Autodesk Fusion 360 part; units mm, degrees
(part 2 of 3)
  line L889 (-65.0001, -30.25) -> (-65.0001, -32.25)
  line L890 (-62.5001, -30.25) -> (-62.5001, -32.25)
  line L891 (-27.5001, -35.25) -> (-27.5001, -37.25)
  line L892 (-32.5001, -39.75) -> (-30.5001, -39.75)
  line L893 (-30.5001, -32.75) -> (-32.5001, -32.75)
  line L894 (-55.5001, -37.25) -> (-55.5001, -35.25)
  line L895 (-32.5001, -32.25) -> (-30.5001, -32.25)
  line L896 (-53.0001, -40.25) -> (-55.0001, -40.25)
  line L897 (-30.5001, -34.75) -> (-30.5001, -32.75)
  line L898 (-30.5001, -32.25) -> (-30.5001, -30.25)
  line L899 (-72.5001, -37.75) -> (-72.5001, -39.75)
  line L900 (-32.5001, -30.25) -> (-32.5001, -32.25)
  line L901 (-28.0001, -37.25) -> (-28.0001, -35.25)
  line L902 (-38.0001, -34.75) -> (-38.0001, -32.75)
  line L903 (-55.0001, -37.25) -> (-53.0001, -37.25)
  line L904 (-55.0001, -37.75) -> (-55.0001, -39.75)
  line L905 (-30.0001, -37.25) -> (-28.0001, -37.25)
  line L906 (-72.5001, -39.75) -> (-70.5001, -39.75)
  line L907 (-15.0001, -37.75) -> (-15.0001, -39.75)
  line L908 (-30.5001, -30.25) -> (-32.5001, -30.25)
  line L909 (-72.5001, -34.75) -> (-70.5001, -34.75)
  line L910 (-53.0001, -30.25) -> (-55.0001, -30.25)
  line L911 (-12.5001, -32.25) -> (-10.5001, -32.25)
  line L912 (-40.5001, -32.75) -> (-42.5001, -32.75)
  line L913 (-53.0001, -42.25) -> (-53.0001, -40.25)
  line L914 (-53.0001, -39.75) -> (-53.0001, -37.75)
  line L915 (-30.0001, -37.75) -> (-30.0001, -39.75)
  line L916 (-55.5001, -42.25) -> (-55.5001, -40.25)
  line L917 (-15.5001, -39.75) -> (-15.5001, -37.75)
  line L918 (-55.0001, -39.75) -> (-53.0001, -39.75)
  line L919 (-53.0001, -35.25) -> (-55.0001, -35.25)
  line L920 (-40.5001, -30.25) -> (-42.5001, -30.25)
  line L921 (-27.5001, -37.75) -> (-27.5001, -39.75)
  line L922 (-72.5001, -37.25) -> (-70.5001, -37.25)
  line L923 (-40.5001, -35.25) -> (-42.5001, -35.25)
  line L924 (-32.5001, -32.75) -> (-32.5001, -34.75)
  line L925 (-30.5001, -35.25) -> (-32.5001, -35.25)
  line L926 (-70.5001, -32.75) -> (-72.5001, -32.75)
  line L927 (-72.5001, -32.25) -> (-70.5001, -32.25)
  line L928 (-53.0001, -37.75) -> (-55.0001, -37.75)
  line L929 (-12.5001, -34.75) -> (-10.5001, -34.75)
  line L930 (-55.0001, -30.25) -> (-55.0001, -32.25)
  line L931 (-40.5001, -32.25) -> (-40.5001, -30.25)
  line L932 (-40.5001, -34.75) -> (-40.5001, -32.75)
  line L933 (-13.0001, -39.75) -> (-13.0001, -37.75)
  line L934 (-72.5001, -32.75) -> (-72.5001, -34.75)
  line L935 (-55.0001, -34.75) -> (-53.0001, -34.75)
  line L936 (-53.0001, -37.25) -> (-53.0001, -35.25)
  line L937 (-32.5001, -34.75) -> (-30.5001, -34.75)
  line L938 (-53.0001, -32.25) -> (-53.0001, -30.25)
  line L939 (-28.0001, -39.75) -> (-28.0001, -37.75)
  line L940 (-30.0001, -35.25) -> (-30.0001, -37.25)
  line L941 (-30.0001, -32.25) -> (-28.0001, -32.25)
  line L942 (-30.0001, -32.75) -> (-30.0001, -34.75)
  line L943 (-40.0001, -32.75) -> (-40.0001, -34.75)
  line L944 (-10.5001, -37.75) -> (-12.5001, -37.75)
  line L945 (-32.5001, -35.25) -> (-32.5001, -37.25)
  line L946 (-30.0001, -30.25) -> (-30.0001, -32.25)
  line L947 (-42.5001, -34.75) -> (-40.5001, -34.75)
  line L948 (-55.0001, -40.25) -> (-55.0001, -42.25)
  line L949 (-55.0001, -42.25) -> (-53.0001, -42.25)
  line L950 (-70.5001, -37.75) -> (-72.5001, -37.75)
  line L951 (-55.5001, -39.75) -> (-55.5001, -37.75)
  line L952 (-55.0001, -35.25) -> (-55.0001, -37.25)
  line L953 (-15.0001, -32.25) -> (-13.0001, -32.25)
  line L954 (-75.5001, -40.25) -> (-77.5001, -40.25)
  line L955 (-53.0001, -34.75) -> (-53.0001, -32.75)
  line L956 (-77.5001, -42.25) -> (-75.5001, -42.25)
  line L957 (-53.0001, -32.75) -> (-55.0001, -32.75)
  line L958 (-78.0001, -42.25) -> (-78.0001, -40.25)
  line L959 (-25.5001, -34.75) -> (-25.5001, -32.75)
  line L960 (-55.5001, -32.25) -> (-55.5001, -30.25)
  line L961 (-67.5001, -32.75) -> (-67.5001, -34.75)
  line L962 (-27.5001, -42.25) -> (-25.5001, -42.25)
  line L963 (-33.0001, -37.25) -> (-33.0001, -35.25)
  line L964 (-40.0001, -32.25) -> (-38.0001, -32.25)
  line L965 (-38.0001, -32.25) -> (-38.0001, -30.25)
  line L966 (-70.0001, -32.75) -> (-70.0001, -34.75)
  line L967 (-55.0001, -32.75) -> (-55.0001, -34.75)
  line L968 (-20.5001, -37.75) -> (-22.5001, -37.75)
  line L969 (-28.0001, -32.25) -> (-28.0001, -30.25)
  line L970 (-13.0001, -30.25) -> (-15.0001, -30.25)
  line L971 (-25.0001, -32.75) -> (-25.0001, -34.75)
  line L972 (-70.5001, -35.25) -> (-72.5001, -35.25)
  line L973 (-55.5001, -34.75) -> (-55.5001, -32.75)
  line L974 (-27.5001, -30.25) -> (-27.5001, -32.25)
  line L975 (-72.5001, -30.25) -> (-72.5001, -32.25)
  line L976 (-13.0001, -32.75) -> (-15.0001, -32.75)
  line L977 (-20.5001, -35.25) -> (-22.5001, -35.25)
  line L978 (-15.0001, -30.25) -> (-15.0001, -32.25)
  line L979 (-35.0001, -42.25) -> (-33.0001, -42.25)
  line L980 (-72.5001, -35.25) -> (-72.5001, -37.25)
  line L981 (-13.0001, -32.25) -> (-13.0001, -30.25)
  line L982 (-12.5001, -32.75) -> (-12.5001, -34.75)
  line L983 (-70.0001, -30.25) -> (-70.0001, -32.25)
  line L984 (-27.5001, -32.75) -> (-27.5001, -34.75)
  line L985 (-40.0001, -30.25) -> (-40.0001, -32.25)
  line L986 (-35.5001, -40.25) -> (-37.5001, -40.25)
  line L987 (-33.0001, -40.25) -> (-35.0001, -40.25)
  line L988 (-28.0001, -34.75) -> (-28.0001, -32.75)
  line L989 (-70.5001, -30.25) -> (-72.5001, -30.25)
  line L990 (-33.0001, -42.25) -> (-33.0001, -40.25)
  line L991 (-37.5001, -40.25) -> (-37.5001, -42.25)
  line L992 (-40.5001, -37.25) -> (-40.5001, -35.25)
  line L993 (-22.5001, -34.75) -> (-20.5001, -34.75)
  line L994 (-37.5001, -42.25) -> (-35.5001, -42.25)
  line L995 (-55.0001, -32.25) -> (-53.0001, -32.25)
  line L996 (-15.5001, -34.75) -> (-15.5001, -32.75)
  line L997 (-30.5001, -37.25) -> (-30.5001, -35.25)
  line L998 (-38.0001, -30.25) -> (-40.0001, -30.25)
  line L999 (-35.5001, -42.25) -> (-35.5001, -40.25)
  line L1000 (-68.0001, -34.75) -> (-68.0001, -32.75)
  line L1001 (-15.5001, -32.25) -> (-15.5001, -30.25)
  line L1002 (-22.5001, -39.75) -> (-20.5001, -39.75)
  line L1003 (-35.0001, -40.25) -> (-35.0001, -42.25)
  line L1004 (-77.5001, -40.25) -> (-77.5001, -42.25)
  line L1005 (-42.5001, -32.25) -> (-40.5001, -32.25)
  line L1006 (-12.5001, -30.25) -> (-12.5001, -32.25)
  line L1007 (-47.5001, -37.75) -> (-47.5001, -39.75)
  line L1008 (-43.0001, -39.75) -> (-43.0001, -37.75)
  line L1009 (-45.0001, -37.75) -> (-45.0001, -39.75)
  line L1010 (-67.5001, -35.25) -> (-67.5001, -37.25)
  line L1011 (-75.5001, -35.25) -> (-77.5001, -35.25)
  line L1012 (-57.5001, -35.25) -> (-57.5001, -37.25)
  line L1013 (-57.5001, -37.25) -> (-55.5001, -37.25)
  line L1014 (-25.5001, -37.75) -> (-27.5001, -37.75)
  line L1015 (-35.0001, -34.75) -> (-33.0001, -34.75)
  line L1016 (-78.0001, -34.75) -> (-78.0001, -32.75)
  line L1017 (-35.5001, -32.25) -> (-35.5001, -30.25)
  line L1018 (-35.5001, -34.75) -> (-35.5001, -32.75)
  line L1019 (-60.0001, -40.25) -> (-60.0001, -42.25)
  line L1020 (-57.5001, -34.75) -> (-55.5001, -34.75)
  line L1021 (-55.5001, -35.25) -> (-57.5001, -35.25)
  line L1022 (-78.0001, -39.75) -> (-78.0001, -37.75)
  line L1023 (-37.5001, -30.25) -> (-37.5001, -32.25)
  line L1024 (-65.5001, -35.25) -> (-67.5001, -35.25)
  line L1025 (-55.5001, -37.75) -> (-57.5001, -37.75)
  line L1026 (-77.5001, -39.75) -> (-75.5001, -39.75)
  line L1027 (-25.5001, -37.25) -> (-25.5001, -35.25)
  line L1028 (-35.5001, -30.25) -> (-37.5001, -30.25)
  line L1029 (-67.5001, -34.75) -> (-65.5001, -34.75)
  line L1030 (-58.0001, -37.75) -> (-60.0001, -37.75)
  line L1031 (-60.0001, -39.75) -> (-58.0001, -39.75)
  line L1032 (-35.5001, -35.25) -> (-37.5001, -35.25)
  line L1033 (-55.5001, -32.75) -> (-57.5001, -32.75)
  line L1034 (-57.5001, -40.25) -> (-57.5001, -42.25)
  line L1035 (-35.0001, -37.75) -> (-35.0001, -39.75)
  line L1036 (-37.5001, -37.25) -> (-35.5001, -37.25)
  line L1037 (-37.5001, -32.75) -> (-37.5001, -34.75)
  line L1038 (-33.0001, -35.25) -> (-35.0001, -35.25)
  line L1039 (-60.0001, -37.25) -> (-58.0001, -37.25)
  line L1040 (-60.5001, -42.25) -> (-60.5001, -40.25)
  line L1041 (-57.5001, -37.75) -> (-57.5001, -39.75)
  line L1042 (-77.5001, -37.75) -> (-77.5001, -39.75)
  line L1043 (-33.0001, -32.75) -> (-35.0001, -32.75)
  line L1044 (-37.5001, -39.75) -> (-35.5001, -39.75)
  line L1045 (-73.0001, -32.75) -> (-75.0001, -32.75)
  line L1046 (-58.0001, -42.25) -> (-58.0001, -40.25)
  line L1047 (-27.5001, -37.25) -> (-25.5001, -37.25)
  line L1048 (-68.0001, -37.25) -> (-68.0001, -35.25)
  line L1049 (-60.5001, -39.75) -> (-60.5001, -37.75)
  line L1050 (-37.5001, -34.75) -> (-35.5001, -34.75)
  line L1051 (-37.5001, -32.25) -> (-35.5001, -32.25)
  line L1052 (-75.0001, -34.75) -> (-73.0001, -34.75)
  line L1053 (-60.0001, -37.75) -> (-60.0001, -39.75)
  line L1054 (-77.5001, -37.25) -> (-75.5001, -37.25)
  line L1055 (-35.5001, -39.75) -> (-35.5001, -37.75)
  line L1056 (-67.5001, -37.25) -> (-65.5001, -37.25)
  line L1057 (-33.0001, -34.75) -> (-33.0001, -32.75)
  line L1058 (-75.5001, -30.25) -> (-77.5001, -30.25)
  line L1059 (-75.0001, -32.75) -> (-75.0001, -34.75)
  line L1060 (-35.0001, -32.75) -> (-35.0001, -34.75)
  line L1061 (-78.0001, -32.25) -> (-78.0001, -30.25)
  line L1062 (-58.0001, -40.25) -> (-60.0001, -40.25)
  line L1063 (-75.5001, -32.75) -> (-77.5001, -32.75)
  line L1064 (-77.5001, -30.25) -> (-77.5001, -32.25)
  line L1065 (-75.5001, -37.75) -> (-77.5001, -37.75)
  line L1066 (-58.0001, -39.75) -> (-58.0001, -37.75)
  line L1067 (-60.0001, -42.25) -> (-58.0001, -42.25)
  line L1068 (-65.5001, -37.75) -> (-67.5001, -37.75)
  line L1069 (-73.0001, -35.25) -> (-75.0001, -35.25)
  line L1070 (-77.5001, -32.25) -> (-75.5001, -32.25)
  line L1071 (-58.0001, -32.25) -> (-58.0001, -30.25)
  line L1072 (-58.0001, -30.25) -> (-60.0001, -30.25)
  line L1073 (-20.0001, -32.25) -> (-18.0001, -32.25)
  line L1074 (-20.0001, -39.75) -> (-18.0001, -39.75)
  line L1075 (-18.0001, -42.25) -> (-18.0001, -40.25)
  line L1076 (-17.5001, -40.25) -> (-17.5001, -42.25)
  line L1077 (-17.5001, -30.25) -> (-17.5001, -32.25)
  line L1078 (-20.5001, -34.75) -> (-20.5001, -32.75)
  line L1079 (-75.0001, -30.25) -> (-75.0001, -32.25)
  line L1080 (-60.5001, -37.25) -> (-60.5001, -35.25)
  line L1081 (-35.0001, -32.25) -> (-33.0001, -32.25)
  line L1082 (-18.0001, -34.75) -> (-18.0001, -32.75)
  line L1083 (-17.5001, -37.75) -> (-17.5001, -39.75)
  line L1084 (-20.5001, -32.25) -> (-20.5001, -30.25)
  line L1085 (-20.0001, -42.25) -> (-18.0001, -42.25)
  line L1086 (-18.0001, -32.75) -> (-20.0001, -32.75)
  line L1087 (-35.0001, -30.25) -> (-35.0001, -32.25)
  line L1088 (-33.0001, -30.25) -> (-35.0001, -30.25)
  line L1089 (-58.0001, -35.25) -> (-60.0001, -35.25)
  line L1090 (-33.0001, -32.25) -> (-33.0001, -30.25)
  line L1091 (-73.0001, -30.25) -> (-75.0001, -30.25)
  line L1092 (-57.5001, -32.25) -> (-55.5001, -32.25)
  line L1093 (-55.5001, -40.25) -> (-57.5001, -40.25)
  line L1094 (-57.5001, -30.25) -> (-57.5001, -32.25)
  line L1095 (-58.0001, -37.25) -> (-58.0001, -35.25)
  line L1096 (-17.5001, -32.75) -> (-17.5001, -34.75)
  line L1097 (-60.0001, -32.25) -> (-58.0001, -32.25)
  line L1098 (-60.5001, -32.25) -> (-60.5001, -30.25)
  line L1099 (-75.0001, -32.25) -> (-73.0001, -32.25)
  line L1100 (-55.5001, -30.25) -> (-57.5001, -30.25)
  line L1101 (-60.0001, -32.75) -> (-60.0001, -34.75)
  line L1102 (-58.0001, -32.75) -> (-60.0001, -32.75)
  line L1103 (-58.0001, -34.75) -> (-58.0001, -32.75)
  line L1104 (-20.0001, -37.75) -> (-20.0001, -39.75)
  line L1105 (-18.0001, -39.75) -> (-18.0001, -37.75)
  line L1106 (-20.5001, -39.75) -> (-20.5001, -37.75)
  line L1107 (-77.5001, -34.75) -> (-75.5001, -34.75)
  line L1108 (-57.5001, -42.25) -> (-55.5001, -42.25)
  line L1109 (-60.0001, -34.75) -> (-58.0001, -34.75)
  line L1110 (-57.5001, -32.75) -> (-57.5001, -34.75)
  line L1111 (-20.0001, -32.75) -> (-20.0001, -34.75)
  line L1112 (-60.5001, -34.75) -> (-60.5001, -32.75)
  line L1113 (-57.5001, -39.75) -> (-55.5001, -39.75)
  line L1114 (-60.0001, -30.25) -> (-60.0001, -32.25)
  line L1115 (-60.0001, -35.25) -> (-60.0001, -37.25)
  line L1116 (-77.5001, -32.75) -> (-77.5001, -34.75)
  line L1117 (-78.0001, -40.25) -> (-80.0001, -40.25)
  line L1118 (-62.5001, -40.25) -> (-62.5001, -42.25)
  line L1119 (-20.5001, -42.25) -> (-20.5001, -40.25)
  line L1120 (-18.0001, -30.25) -> (-20.0001, -30.25)
  line L1121 (-75.5001, -34.75) -> (-75.5001, -32.75)
  line L1122 (-65.5001, -42.25) -> (-65.5001, -40.25)
  line L1123 (-75.5001, -42.25) -> (-75.5001, -40.25)
  line L1124 (-65.0001, -42.25) -> (-63.0001, -42.25)
  line L1125 (-17.5001, -35.25) -> (-17.5001, -37.25)
  line L1126 (-20.0001, -37.25) -> (-18.0001, -37.25)
  line L1127 (-70.0001, -37.75) -> (-70.0001, -39.75)
  line L1128 (-20.0001, -30.25) -> (-20.0001, -32.25)
  line L1129 (-75.5001, -39.75) -> (-75.5001, -37.75)
  line L1130 (-18.0001, -35.25) -> (-20.0001, -35.25)
  line L1131 (-73.0001, -37.75) -> (-75.0001, -37.75)
  line L1132 (-18.0001, -37.25) -> (-18.0001, -35.25)
  line L1133 (-20.5001, -37.25) -> (-20.5001, -35.25)
  line L1134 (-68.0001, -40.25) -> (-70.0001, -40.25)
  line L1135 (-75.0001, -40.25) -> (-75.0001, -42.25)
  line L1136 (-80.0001, -32.75) -> (-80.0001, -34.75)
  line L1137 (-70.0001, -40.25) -> (-70.0001, -42.25)
  line L1138 (-70.0001, -37.25) -> (-68.0001, -37.25)
  line L1139 (-75.0001, -42.25) -> (-73.0001, -42.25)
  line L1140 (-70.5001, -42.25) -> (-70.5001, -40.25)
  line L1141 (-20.0001, -34.75) -> (-18.0001, -34.75)
  line L1142 (-18.0001, -32.25) -> (-18.0001, -30.25)
  line L1143 (-73.0001, -40.25) -> (-75.0001, -40.25)
  line L1144 (-18.0001, -40.25) -> (-20.0001, -40.25)
  line L1145 (-73.0001, -39.75) -> (-73.0001, -37.75)
  line L1146 (-18.0001, -37.75) -> (-20.0001, -37.75)
  line L1147 (-80.0001, -39.75) -> (-78.0001, -39.75)
  line L1148 (-73.0001, -42.25) -> (-73.0001, -40.25)
  line L1149 (-63.0001, -40.25) -> (-65.0001, -40.25)
  line L1150 (-70.0001, -42.25) -> (-68.0001, -42.25)
  line L1151 (-20.0001, -40.25) -> (-20.0001, -42.25)
  line L1152 (-73.0001, -32.25) -> (-73.0001, -30.25)
  line L1153 (-20.0001, -35.25) -> (-20.0001, -37.25)
  line L1154 (-70.0001, -39.75) -> (-68.0001, -39.75)
  line L1155 (-80.0001, -37.75) -> (-80.0001, -39.75)
  line L1156 (-63.0001, -42.25) -> (-63.0001, -40.25)
  line L1157 (-70.5001, -39.75) -> (-70.5001, -37.75)
  line L1158 (-80.0001, -40.25) -> (-80.0001, -42.25)
  line L1159 (-65.0001, -40.25) -> (-65.0001, -42.25)
  line L1160 (-75.0001, -37.25) -> (-73.0001, -37.25)
  line L1161 (-75.0001, -39.75) -> (-73.0001, -39.75)
  line L1162 (-80.0001, -42.25) -> (-78.0001, -42.25)
  line L1163 (-75.0001, -37.75) -> (-75.0001, -39.75)
  line L1164 (-78.0001, -37.25) -> (-78.0001, -35.25)
  line L1165 (-35.0001, -35.25) -> (-35.0001, -37.25)
  line L1166 (-68.0001, -42.25) -> (-68.0001, -40.25)
  line L1167 (-27.5001, -32.25) -> (-25.5001, -32.25)
  line L1168 (-65.5001, -30.25) -> (-67.5001, -30.25)
  line L1169 (-77.5001, -35.25) -> (-77.5001, -37.25)
  line L1170 (-37.5001, -37.75) -> (-37.5001, -39.75)
  line L1171 (-25.5001, -40.25) -> (-27.5001, -40.25)
  line L1172 (-25.0001, -37.75) -> (-25.0001, -39.75)
  line L1173 (-27.5001, -39.75) -> (-25.5001, -39.75)
  line L1174 (-35.0001, -37.25) -> (-33.0001, -37.25)
  line L1175 (-65.5001, -32.75) -> (-67.5001, -32.75)
  line L1176 (-68.0001, -32.25) -> (-68.0001, -30.25)
  line L1177 (-67.5001, -40.25) -> (-67.5001, -42.25)
  line L1178 (-67.5001, -32.25) -> (-65.5001, -32.25)
  line L1179 (-67.5001, -30.25) -> (-67.5001, -32.25)
  line L1180 (-35.0001, -39.75) -> (-33.0001, -39.75)
  line L1181 (-35.5001, -37.75) -> (-37.5001, -37.75)
  line L1182 (-67.5001, -37.75) -> (-67.5001, -39.75)
  line L1183 (-25.5001, -32.75) -> (-27.5001, -32.75)
  line L1184 (-25.0001, -30.25) -> (-25.0001, -32.25)
  line L1185 (-25.5001, -42.25) -> (-25.5001, -40.25)
  line L1186 (-67.5001, -39.75) -> (-65.5001, -39.75)
  line L1187 (-35.5001, -37.25) -> (-35.5001, -35.25)
  line L1188 (-25.0001, -35.25) -> (-25.0001, -37.25)
  line L1189 (-35.5001, -32.75) -> (-37.5001, -32.75)
  line L1190 (-33.0001, -37.75) -> (-35.0001, -37.75)
  line L1191 (-65.5001, -40.25) -> (-67.5001, -40.25)
  line L1192 (-25.5001, -35.25) -> (-27.5001, -35.25)
  line L1193 (-27.5001, -34.75) -> (-25.5001, -34.75)
  line L1194 (-25.5001, -39.75) -> (-25.5001, -37.75)
  line L1195 (-33.0001, -39.75) -> (-33.0001, -37.75)
  line L1196 (-25.5001, -30.25) -> (-27.5001, -30.25)
  line L1197 (-67.5001, -42.25) -> (-65.5001, -42.25)
  line L1198 (-25.5001, -32.25) -> (-25.5001, -30.25)
  line L1199 (-37.5001, -35.25) -> (-37.5001, -37.25)
  line L1200 (-68.0001, -39.75) -> (-68.0001, -37.75)
  line L1201 (-25.0001, -40.25) -> (-25.0001, -42.25)
  line L1202 (-43.0001, -35.25) -> (-45.0001, -35.25)
  line L1203 (-50.0001, -34.75) -> (-48.0001, -34.75)
  line L1204 (-48.0001, -37.75) -> (-50.0001, -37.75)
  line L1205 (-50.5001, -37.25) -> (-50.5001, -35.25)
  line L1206 (-42.5001, -32.75) -> (-42.5001, -34.75)
  line L1207 (-50.5001, -39.75) -> (-50.5001, -37.75)
  line L1208 (-45.5001, -39.75) -> (-45.5001, -37.75)
  line L1209 (-50.0001, -37.25) -> (-48.0001, -37.25)
  line L1210 (-50.0001, -35.25) -> (-50.0001, -37.25)
  line L1211 (-48.0001, -35.25) -> (-50.0001, -35.25)
  line L1212 (-45.0001, -34.75) -> (-43.0001, -34.75)
  line L1213 (-45.0001, -37.25) -> (-43.0001, -37.25)
  line L1214 (-43.0001, -37.25) -> (-43.0001, -35.25)
  line L1215 (-45.5001, -35.25) -> (-47.5001, -35.25)
  line L1216 (-45.5001, -37.25) -> (-45.5001, -35.25)
  line L1217 (-42.5001, -35.25) -> (-42.5001, -37.25)
  line L1218 (-47.5001, -37.25) -> (-45.5001, -37.25)
  line L1219 (-47.5001, -35.25) -> (-47.5001, -37.25)
  line L1220 (-48.0001, -37.25) -> (-48.0001, -35.25)
  line L1221 (-50.0001, -37.75) -> (-50.0001, -39.75)
  line L1222 (-48.0001, -39.75) -> (-48.0001, -37.75)
  line L1223 (-47.5001, -30.25) -> (-47.5001, -32.25)
  line L1224 (-48.0001, -34.75) -> (-48.0001, -32.75)
  line L1225 (-50.0001, -32.75) -> (-50.0001, -34.75)
  line L1226 (-50.5001, -34.75) -> (-50.5001, -32.75)
  line L1227 (-50.0001, -32.25) -> (-48.0001, -32.25)
  line L1228 (-45.0001, -30.25) -> (-45.0001, -32.25)
  line L1229 (-43.0001, -34.75) -> (-43.0001, -32.75)
  line L1230 (-43.0001, -32.25) -> (-43.0001, -30.25)
  line L1231 (-45.0001, -32.25) -> (-43.0001, -32.25)
  line L1232 (-45.5001, -32.25) -> (-45.5001, -30.25)
  line L1233 (-50.5001, -32.25) -> (-50.5001, -30.25)
  line L1234 (-45.5001, -32.75) -> (-47.5001, -32.75)
  line L1235 (-48.0001, -32.25) -> (-48.0001, -30.25)
  line L1236 (-45.5001, -30.25) -> (-47.5001, -30.25)
  line L1237 (-43.0001, -32.75) -> (-45.0001, -32.75)
  line L1238 (-48.0001, -32.75) -> (-50.0001, -32.75)
  line L1239 (-43.0001, -30.25) -> (-45.0001, -30.25)
  line L1240 (-47.5001, -32.25) -> (-45.5001, -32.25)
  line L1241 (-50.0001, -30.25) -> (-50.0001, -32.25)
  line L1242 (-48.0001, -30.25) -> (-50.0001, -30.25)
  line L1243 (-42.5001, -30.25) -> (-42.5001, -32.25)
  line L1244 (-47.5001, -32.75) -> (-47.5001, -34.75)
  line L1245 (-45.5001, -34.75) -> (-45.5001, -32.75)
  dimension "d443" = 3.0001
  dimension "d445" = 2.9999
  dimension "d446" = 1.75
  constraint horizontal L9
  constraint vertical L6
  constraint horizontal L7
  constraint vertical L8
  constraint horizontal L10
  constraint vertical L11
  constraint horizontal L12
  constraint vertical L13
  constraint horizontal L16
  constraint vertical L17
  constraint horizontal L14
  constraint vertical L15
  constraint horizontal L21
  constraint vertical L20
  constraint horizontal L18
  constraint vertical L19
  constraint horizontal L24
  constraint vertical L25
  constraint horizontal L22
  constraint vertical L23
  constraint horizontal L32
  constraint vertical L26
  constraint horizontal L33
  constraint vertical L29
  constraint horizontal L39
  constraint vertical L43
  constraint horizontal L41
  constraint vertical L40
  constraint horizontal L37
  constraint vertical L42
  constraint horizontal L38
  constraint vertical L35
  constraint horizontal L28
  constraint vertical L34
  constraint horizontal L45
  constraint vertical L27
  constraint horizontal L36
  constraint vertical L31
  constraint horizontal L30
  constraint vertical L44
  constraint horizontal L60
  constraint vertical L61
  constraint horizontal L84
  constraint vertical L81
  constraint horizontal L66
  constraint vertical L72
  constraint horizontal L85
  constraint vertical L64
  constraint horizontal L51
  constraint vertical L65
  constraint horizontal L58
  constraint vertical L47
  constraint horizontal L62
  constraint vertical L68
  constraint horizontal L63
  constraint vertical L71
  constraint horizontal L55
  constraint vertical L73
  constraint horizontal L78
  constraint vertical L79
  constraint horizontal L49
  constraint vertical L46
  constraint horizontal L80
  constraint vertical L57
  constraint horizontal L69
  constraint vertical L67
  constraint horizontal L59
  constraint vertical L56
  constraint horizontal L50
  constraint vertical L54
  constraint horizontal L76
  constraint vertical L48
  constraint horizontal L77
  constraint vertical L83
  constraint horizontal L75
  constraint vertical L82
  constraint horizontal L70
  constraint vertical L53
  constraint horizontal L74
  constraint vertical L52
  constraint horizontal L89
  constraint vertical L151
  constraint horizontal L102
  constraint vertical L86
  constraint horizontal L155
  constraint vertical L164
  constraint horizontal L109
  constraint vertical L146
  constraint horizontal L145
  constraint vertical L108
  constraint horizontal L91
  constraint vertical L126
  constraint horizontal L95
  constraint vertical L152
  constraint horizontal L103
  constraint vertical L100
  constraint horizontal L101
  constraint vertical L88
  constraint horizontal L99
  constraint vertical L96
  constraint horizontal L156
  constraint vertical L122
  constraint horizontal L147
  constraint vertical L90
  constraint horizontal L150
  constraint vertical L87
  constraint horizontal L148
  constraint vertical L98
  constraint horizontal L133
  constraint vertical L104
  constraint horizontal L163
  constraint vertical L123
  constraint horizontal L94
  constraint vertical L143
  constraint horizontal L160
  constraint vertical L92
  constraint horizontal L134
  constraint vertical L107
  constraint horizontal L153
  constraint vertical L97
  constraint horizontal L105
  constraint vertical L119
  constraint horizontal L131
  constraint vertical L110
  constraint horizontal L154
  constraint vertical L132
  constraint horizontal L162
  constraint vertical L93
  constraint horizontal L149
  constraint vertical L124
  constraint horizontal L140
  constraint vertical L125
  constraint horizontal L139
  constraint vertical L135
  constraint horizontal L137
  constraint vertical L142
  constraint horizontal L106
  constraint vertical L113
  constraint horizontal L111
  constraint vertical L114
  constraint horizontal L120
  constraint vertical L121
  constraint horizontal L128
  constraint vertical L118
  constraint horizontal L136
  constraint vertical L138
  constraint horizontal L127
  constraint vertical L141
  constraint horizontal L115
  constraint vertical L112
  constraint horizontal L157
  constraint vertical L159
  constraint horizontal L116
  constraint vertical L158
  constraint horizontal L165
  constraint vertical L161
  constraint horizontal L130
  constraint vertical L117
  constraint horizontal L129
  constraint vertical L144
  constraint horizontal L320
  constraint vertical L323
  constraint horizontal L194
  constraint vertical L317
  constraint horizontal L302
  constraint vertical L247
  constraint horizontal L214
  constraint vertical L284
  constraint horizontal L266
  constraint vertical L233
  constraint horizontal L283
  constraint vertical L248
  constraint horizontal L306
  constraint vertical L290
  constraint horizontal L197
  constraint vertical L309
  constraint horizontal L319
  constraint vertical L325
  constraint horizontal L295
  constraint vertical L316
  constraint horizontal L230
  constraint vertical L282
  constraint horizontal L244
  constraint vertical L324
  constraint horizontal L265
  constraint vertical L225
  constraint horizontal L308
  constraint vertical L293
  constraint horizontal L297
  constraint vertical L187
  constraint horizontal L270
  constraint vertical L259
  constraint horizontal L239
  constraint vertical L231
  constraint horizontal L226
  constraint vertical L288
  constraint horizontal L246
  constraint vertical L278
  constraint horizontal L289
  constraint vertical L313
  constraint horizontal L298
  constraint vertical L281
  constraint horizontal L280
  constraint vertical L291
  constraint horizontal L274
  constraint vertical L237
  constraint horizontal L262
  constraint vertical L240
  constraint horizontal L251
  constraint vertical L241
  constraint horizontal L261
  constraint vertical L269
  constraint horizontal L222
  constraint vertical L238
  constraint horizontal L264
  constraint vertical L263
  constraint horizontal L287
  constraint vertical L305
  constraint horizontal L294
  constraint vertical L310
  constraint horizontal L277
  constraint vertical L227
  constraint horizontal L299
  constraint vertical L236
  constraint horizontal L258
  constraint vertical L220
  constraint horizontal L252
  constraint vertical L250
  constraint horizontal L243
  constraint vertical L216
  constraint horizontal L249
  constraint vertical L322
  constraint horizontal L271
  constraint vertical L268
  constraint horizontal L245
  constraint vertical L321
  constraint horizontal L275
  constraint vertical L307
  constraint horizontal L312
  constraint vertical L276
  constraint horizontal L279
  constraint vertical L253
  constraint horizontal L229
  constraint vertical L255
  constraint horizontal L267
  constraint vertical L221
  constraint horizontal L234
  constraint vertical L260
  constraint horizontal L228
  constraint vertical L303
  constraint horizontal L300
  constraint vertical L296
  constraint horizontal L314
  constraint vertical L301
  constraint horizontal L318
  constraint vertical L315
  constraint horizontal L285
  constraint vertical L286
  constraint horizontal L292
  constraint vertical L311
  constraint horizontal L198
  constraint vertical L217
  constraint horizontal L178
  constraint vertical L254
  constraint horizontal L175
  constraint vertical L169
  constraint horizontal L177
  constraint vertical L181
  constraint horizontal L176
  constraint vertical L196
  constraint horizontal L213
  constraint vertical L186
  constraint horizontal L192
  constraint vertical L210
  constraint horizontal L195
  constraint vertical L232
  constraint horizontal L188
  constraint vertical L242
  constraint horizontal L191
  constraint vertical L304
  constraint horizontal L224
  constraint vertical L208
  constraint horizontal L173
  constraint vertical L209
  constraint horizontal L180
  constraint vertical L171
  constraint horizontal L174
  constraint vertical L182
  constraint horizontal L167
  constraint vertical L189
  constraint horizontal L200
  constraint vertical L206
  constraint horizontal L185
  constraint vertical L219
  constraint horizontal L204
  constraint vertical L199
  constraint horizontal L257
  constraint vertical L272
  constraint horizontal L223
  constraint vertical L273
  constraint horizontal L203
  constraint vertical L215
  constraint horizontal L168
  constraint vertical L212
  constraint horizontal L170
  constraint vertical L183
  constraint horizontal L179
  constraint vertical L166
  constraint horizontal L172
  constraint vertical L202
  constraint horizontal L190
  constraint vertical L218
  constraint horizontal L211
  constraint vertical L184
  constraint horizontal L201
  constraint vertical L205
  constraint horizontal L193
  constraint vertical L256
  constraint horizontal L207
  constraint vertical L235
  constraint horizontal L478
  constraint vertical L458
  constraint horizontal L624
  constraint vertical L495
  constraint horizontal L498
  constraint vertical L525
  constraint horizontal L374
  constraint vertical L578
  constraint horizontal L559
  constraint vertical L397
  constraint horizontal L541
  constraint vertical L389
  constraint horizontal L524
  constraint vertical L564
  constraint horizontal L362
  constraint vertical L565
  constraint horizontal L496
  constraint vertical L470
  constraint horizontal L482
  constraint vertical L457
  constraint horizontal L506
  constraint vertical L504
  constraint horizontal L453
  constraint vertical L479
  constraint horizontal L456
  constraint vertical L530
  constraint horizontal L551
  constraint vertical L556
  constraint horizontal L546
  constraint vertical L370
  constraint horizontal L540
  constraint vertical L480
  constraint horizontal L532
  constraint vertical L466
  constraint horizontal L557
  constraint vertical L536
  constraint horizontal L395
  constraint vertical L475
  constraint horizontal L452
  constraint vertical L491
  constraint horizontal L490
  constraint vertical L454
  constraint horizontal L455
  constraint vertical L481
  constraint horizontal L501
  constraint vertical L516
  constraint horizontal L517
  constraint vertical L522
  constraint horizontal L547
  constraint vertical L416
  constraint horizontal L509
  constraint vertical L442
  constraint horizontal L472
  constraint vertical L510
  constraint horizontal L464
  constraint vertical L483
  constraint horizontal L393
  constraint vertical L392
  constraint horizontal L476
  constraint vertical L485
  constraint horizontal L398
  constraint vertical L459
  constraint horizontal L471
  constraint vertical L450
  constraint horizontal L441
  constraint vertical L507
  constraint horizontal L446
  constraint vertical L545
  constraint horizontal L609
  constraint vertical L361
  constraint horizontal L417
  constraint vertical L548
  constraint horizontal L523
  constraint vertical L520
  constraint horizontal L360
  constraint vertical L544
  constraint horizontal L444
  constraint vertical L420
  constraint horizontal L415
  constraint vertical L433
  constraint horizontal L405
  constraint vertical L591
  constraint horizontal L503
  constraint vertical L489
  constraint horizontal L467
  constraint vertical L473
  constraint horizontal L543
  constraint vertical L449
  constraint horizontal L558
  constraint vertical L531
  constraint horizontal L550
  constraint vertical L562
  constraint horizontal L512
  constraint vertical L542
  constraint horizontal L537
  constraint vertical L561
  constraint horizontal L438
  constraint vertical L401
  constraint horizontal L400
  constraint vertical L404
  constraint horizontal L617
  constraint vertical L499
  constraint horizontal L616
  constraint vertical L584
  constraint horizontal L615
  constraint vertical L519
  constraint horizontal L620
  constraint vertical L538
  constraint horizontal L613
  constraint vertical L602
  constraint horizontal L621
  constraint vertical L528
  constraint horizontal L619
  constraint vertical L573
  constraint horizontal L618
  constraint vertical L566
  constraint horizontal L622
  constraint vertical L497
  constraint horizontal L614
  constraint vertical L424
  constraint horizontal L549
  constraint vertical L474
  constraint horizontal L533
  constraint vertical L477
  constraint horizontal L518
  constraint vertical L555
  constraint horizontal L560
  constraint vertical L515
  constraint horizontal L514
  constraint vertical L607
  constraint horizontal L593
  constraint vertical L580
  constraint horizontal L581
  constraint vertical L569
  constraint horizontal L603
  constraint vertical L583
  constraint horizontal L461
  constraint vertical L448
  constraint horizontal L502
  constraint vertical L465
  constraint horizontal L388
  constraint vertical L427
  constraint horizontal L434
  constraint vertical L579
  constraint horizontal L439
  constraint vertical L436
  constraint horizontal L422
  constraint vertical L526
  constraint horizontal L431
  constraint vertical L408
  constraint horizontal L394
  constraint vertical L599
  constraint horizontal L414
  constraint vertical L403
  constraint horizontal L407
  constraint vertical L572
  constraint horizontal L386
  constraint vertical L421
  constraint horizontal L430
  constraint vertical L468
  constraint horizontal L376
  constraint vertical L568
  constraint horizontal L364
  constraint vertical L426
  constraint horizontal L625
  constraint vertical L354
  constraint horizontal L369
  constraint vertical L425
  constraint horizontal L380
  constraint vertical L350
  constraint horizontal L371
  constraint vertical L440
  constraint horizontal L363
  constraint vertical L355
  constraint horizontal L382
  constraint vertical L443
  constraint horizontal L359
  constraint vertical L592
  constraint horizontal L367
  constraint vertical L432
  constraint horizontal L595
  constraint vertical L513
  constraint horizontal L351
  constraint vertical L605
  constraint horizontal L358
  constraint vertical L585
  constraint horizontal L349
  constraint vertical L353
  constraint horizontal L352
  constraint vertical L577
  constraint horizontal L348
  constraint vertical L575
  constraint horizontal L357
  constraint vertical L571
  constraint horizontal L356
  constraint vertical L347
  constraint horizontal L587
  constraint vertical L511
  constraint horizontal L594
  constraint vertical L589
  constraint horizontal L418
  constraint vertical L399
  constraint horizontal L445
  constraint vertical L539
  constraint horizontal L391
  constraint vertical L610
  constraint horizontal L413
  constraint vertical L576
  constraint horizontal L488
  constraint vertical L563
  constraint horizontal L600
  constraint vertical L582
  constraint horizontal L447
  constraint vertical L608
  constraint horizontal L429
  constraint vertical L604
  constraint horizontal L419
  constraint vertical L435
  constraint horizontal L423
  constraint vertical L521
  constraint horizontal L493
  constraint vertical L333
  constraint horizontal L484
  constraint vertical L460
  constraint horizontal L487
  constraint vertical L368
  constraint horizontal L552
  constraint vertical L570
  constraint horizontal L567
  constraint vertical L385
  constraint horizontal L553
  constraint vertical L534
  constraint horizontal L611
  constraint vertical L390
  constraint horizontal L586
  constraint vertical L598
  constraint horizontal L508
  constraint vertical L336
  constraint horizontal L505
  constraint vertical L500
  constraint horizontal L334
  constraint vertical L612
  constraint horizontal L335
  constraint vertical L337
  constraint horizontal L326
  constraint vertical L462
  constraint horizontal L372
  constraint vertical L384
  constraint horizontal L365
  constraint vertical L377
  constraint horizontal L373
  constraint vertical L623
  constraint horizontal L437
  constraint vertical L410
  constraint horizontal L387
  constraint vertical L428
  constraint horizontal L328
  constraint vertical L329
  constraint horizontal L332
  constraint vertical L330
  constraint horizontal L344
  constraint vertical L338
  constraint horizontal L346
  constraint vertical L345
  constraint horizontal L331
  constraint vertical L492
  constraint horizontal L379
  constraint vertical L463
  constraint horizontal L381
  constraint vertical L383
  constraint horizontal L378
  constraint vertical L366
  constraint horizontal L406
  constraint vertical L409
  constraint horizontal L402
  constraint vertical L411
  constraint horizontal L341
  constraint vertical L342
  constraint horizontal L327
  constraint vertical L343
  constraint horizontal L469
  constraint vertical L527
  constraint horizontal L494
  constraint vertical L340
  constraint horizontal L597
  constraint vertical L606
  constraint horizontal L601
  constraint vertical L451
  constraint horizontal L396
  constraint vertical L590
  constraint horizontal L574
  constraint vertical L375
  constraint horizontal L588
  constraint vertical L596
  constraint horizontal L486
  constraint vertical L412
  constraint horizontal L529
  constraint vertical L554
  constraint horizontal L535
  constraint vertical L339
  constraint horizontal L799
  constraint vertical L743
  constraint horizontal L637
  constraint vertical L710
  constraint horizontal L762
  constraint vertical L651
  constraint horizontal L677
  constraint vertical L785
  constraint horizontal L639
  constraint vertical L636
  constraint horizontal L815
  constraint vertical L659
  constraint horizontal L817
  constraint vertical L679
  constraint horizontal L655
  constraint vertical L790
  constraint horizontal L751
  constraint vertical L737
  constraint horizontal L721
  constraint vertical L709
  constraint horizontal L753
  constraint vertical L804
  constraint horizontal L739
  constraint vertical L713
  constraint horizontal L719
  constraint vertical L668
  constraint horizontal L645
  constraint vertical L793
  constraint horizontal L648
  constraint vertical L680
  constraint horizontal L657
  constraint vertical L662
  constraint horizontal L805
  constraint vertical L658
  constraint horizontal L633
  constraint vertical L638
  constraint horizontal L767
  constraint vertical L735
  constraint horizontal L734
  constraint vertical L755
  constraint horizontal L760
  constraint vertical L744
  constraint horizontal L759
  constraint vertical L711
  constraint horizontal L757
  constraint vertical L660
  constraint horizontal L673
  constraint vertical L675
  constraint horizontal L661
  constraint vertical L650
  constraint horizontal L678
  constraint vertical L632
  constraint horizontal L788
  constraint vertical L784
  constraint horizontal L647
  constraint vertical L640
  constraint horizontal L789
  constraint vertical L825
  constraint horizontal L756
  constraint vertical L771
  constraint horizontal L810
  constraint vertical L982
  constraint horizontal L929
  constraint vertical L750
  constraint horizontal L809
  constraint vertical L725
  constraint horizontal L742
  constraint vertical L643
  constraint horizontal L944
  constraint vertical L808
  constraint horizontal L795
  constraint vertical L672
  constraint horizontal L783
  constraint vertical L818
  constraint horizontal L802
  constraint vertical L671
  constraint horizontal L766
  constraint vertical L1006
  constraint horizontal L911
  constraint vertical L717
  constraint horizontal L976
  constraint vertical L745
  constraint horizontal L723
  constraint vertical L758
  constraint horizontal L747
  constraint vertical L718
  constraint horizontal L708
  constraint vertical L764
  constraint horizontal L722
  constraint vertical L907
  constraint horizontal L791
  constraint vertical L933
  constraint horizontal L777
  constraint vertical L798
  constraint horizontal L787
  constraint vertical L786
  constraint horizontal L970
  constraint vertical L978
  constraint horizontal L953
  constraint vertical L981
  constraint horizontal L674
  constraint vertical L1096
  constraint horizontal L646
  constraint vertical L996
  constraint horizontal L649
  constraint vertical L1125
  constraint horizontal L654
  constraint vertical L726
  constraint horizontal L664
  constraint vertical L1083
  constraint horizontal L669
  constraint vertical L917
  constraint horizontal L665
  constraint vertical L1076
  constraint horizontal L652
  constraint vertical L823
  constraint horizontal L653
  constraint vertical L1077
  constraint horizontal L676
  constraint vertical L1001
  constraint horizontal L1086
  constraint vertical L1111
  constraint horizontal L1141
  constraint vertical L1082
  constraint horizontal L1130
  constraint vertical L1153
  constraint horizontal L1126
  constraint vertical L1132
  constraint horizontal L1146
  constraint vertical L1104
  constraint horizontal L1074
  constraint vertical L1105
  constraint horizontal L1144
  constraint vertical L1151
  constraint horizontal L1085
  constraint vertical L1075
  constraint horizontal L1120
  constraint vertical L1128
  constraint horizontal L1073
  constraint vertical L1142
  constraint horizontal L820
  constraint vertical L782
  constraint horizontal L993
  constraint vertical L1078
  constraint horizontal L977
  constraint vertical L781
  constraint horizontal L773
  constraint vertical L1133
  constraint horizontal L968
  constraint vertical L826
  constraint horizontal L1002
  constraint vertical L1106
  constraint horizontal L780
  constraint vertical L816
  constraint horizontal L768
  constraint vertical L1119
  constraint horizontal L800
  constraint vertical L797
  constraint horizontal L761
  constraint vertical L1084
  constraint horizontal L667
  constraint vertical L971
  constraint horizontal L663
  constraint vertical L819
  constraint horizontal L644
  constraint vertical L1188
  constraint horizontal L634
  constraint vertical L821
  constraint horizontal L635
  constraint vertical L1172
  constraint horizontal L641
  constraint vertical L779
  constraint horizontal L666
  constraint vertical L1201
  constraint horizontal L656
  constraint vertical L794
  constraint horizontal L670
  constraint vertical L1184
  constraint horizontal L642
  constraint vertical L814
  constraint horizontal L1183
  constraint vertical L984
  constraint horizontal L1193
  constraint vertical L959
  constraint horizontal L1192
  constraint vertical L891
  constraint horizontal L1047
  constraint vertical L1027
  constraint horizontal L1014
  constraint vertical L921
  constraint horizontal L1173
  constraint vertical L1194
  constraint horizontal L1171
  constraint vertical L807
  constraint horizontal L962
  constraint vertical L1185
  constraint horizontal L1196
  constraint vertical L974
  constraint horizontal L1167
  constraint vertical L1198
  constraint horizontal L727
  constraint vertical L942
  constraint horizontal L714
  constraint vertical L988
  constraint horizontal L724
  constraint vertical L940
  constraint horizontal L905
  constraint vertical L901
  constraint horizontal L716
  constraint vertical L915
  constraint horizontal L774
  constraint vertical L939
  constraint horizontal L770
  constraint vertical L811
  constraint horizontal L813
  constraint vertical L730
  constraint horizontal L775
  constraint vertical L946
  constraint horizontal L941
  constraint vertical L969
  constraint horizontal L893
  constraint vertical L924
  constraint horizontal L937
  constraint vertical L897
  constraint horizontal L925
  constraint vertical L945
  constraint horizontal L728
  constraint vertical L997
  constraint horizontal L720
  constraint vertical L732
  constraint horizontal L892
  constraint vertical L765
  constraint horizontal L792
  constraint vertical L778
  constraint horizontal L776
  constraint vertical L806
  constraint horizontal L908
  constraint vertical L900
  constraint horizontal L895
  constraint vertical L898
  constraint horizontal L1043
  constraint vertical L1060
  constraint horizontal L1015
  constraint vertical L1057
  constraint horizontal L1038
  constraint vertical L1165
  constraint horizontal L1174
  constraint vertical L963
  constraint horizontal L1190
  constraint vertical L1035
  constraint horizontal L1180
  constraint vertical L1195
  constraint horizontal L987
  constraint vertical L1003
  constraint horizontal L979
  constraint vertical L990
  constraint horizontal L1088
  constraint vertical L1087
  constraint horizontal L1081
  constraint vertical L1090
  constraint horizontal L1189
  constraint vertical L1037
  constraint horizontal L1050
  constraint vertical L1018
  constraint horizontal L1032
  constraint vertical L1199
  constraint horizontal L1036
  constraint vertical L1187
  constraint horizontal L1181
  constraint vertical L1170
  constraint horizontal L1044
  constraint vertical L1055
  constraint horizontal L986
  constraint vertical L991
  constraint horizontal L994
  constraint vertical L999
  constraint horizontal L1028
  constraint vertical L1023
  constraint horizontal L1051
  constraint vertical L1017
  constraint horizontal L736
  constraint vertical L943
  constraint horizontal L803
  constraint vertical L902
  constraint horizontal L738
  constraint vertical L748
  constraint horizontal L763
  constraint vertical L741
  constraint horizontal L712
  constraint vertical L715
  constraint horizontal L731
  constraint vertical L752
  constraint horizontal L729
  constraint vertical L746
  constraint horizontal L754
  constraint vertical L740
  constraint horizontal L998
  constraint vertical L985
  constraint horizontal L964
  constraint vertical L965
  constraint horizontal L912
  constraint vertical L1206
  constraint horizontal L947
  constraint vertical L932
  constraint horizontal L923
  constraint vertical L1217
  constraint horizontal L749
  constraint vertical L992
  constraint horizontal L801
  constraint vertical L828
  constraint horizontal L812
  constraint vertical L827
  constraint horizontal L733
  constraint vertical L628
  constraint horizontal L769
  constraint vertical L772
  constraint horizontal L920
  constraint vertical L1243
  constraint horizontal L1005
  constraint vertical L931
  constraint horizontal L1237
  constraint vertical L693
  constraint horizontal L1212
  constraint vertical L1229
  constraint horizontal L1202
  constraint vertical L829
  constraint horizontal L1213
  constraint vertical L1214
  constraint horizontal L832
  constraint vertical L1009
  constraint horizontal L703
  constraint vertical L1008
  constraint horizontal L702
  constraint vertical L698
  constraint horizontal L630
  constraint vertical L707
  constraint horizontal L1239
  constraint vertical L1228
  constraint horizontal L1231
  constraint vertical L1230
  constraint horizontal L1234
  constraint vertical L1244
  constraint horizontal L831
  constraint vertical L1245
  constraint horizontal L1215
  constraint vertical L1219
  constraint horizontal L1218
  constraint vertical L1216
  constraint horizontal L830
  constraint vertical L1007
  constraint horizontal L699
  constraint vertical L1208
  constraint horizontal L631
  constraint vertical L705
  constraint horizontal L700
  constraint vertical L706
  constraint horizontal L1236
  constraint vertical L1223
  constraint horizontal L1240
  constraint vertical L1232
  constraint horizontal L1238
  constraint vertical L1225
  constraint horizontal L1203
  constraint vertical L1224
  constraint horizontal L1211
  constraint vertical L1210
  constraint horizontal L1209
  constraint vertical L1220
  constraint horizontal L1204
  constraint vertical L1221
  constraint horizontal L627
  constraint vertical L1222
  constraint horizontal L704
  constraint vertical L701
  constraint horizontal L697
  constraint vertical L626
  constraint horizontal L1242
  constraint vertical L1241
  constraint horizontal L1227
  constraint vertical L1235
  constraint horizontal L689
  constraint vertical L691
  constraint horizontal L685
  constraint vertical L1226
  constraint horizontal L683
  constraint vertical L692
  constraint horizontal L690
  constraint vertical L1205
  constraint horizontal L688
  constraint vertical L694
  constraint horizontal L687
  constraint vertical L1207
  constraint horizontal L682
  constraint vertical L695
  constraint horizontal L686
  constraint vertical L629
  constraint horizontal L681
  constraint vertical L696
  constraint horizontal L684
  constraint vertical L1233
  constraint horizontal L957
  constraint vertical L967
  constraint horizontal L935
  constraint vertical L955
  constraint horizontal L919
  constraint vertical L952
  constraint horizontal L903
  constraint vertical L936
  constraint horizontal L928
  constraint vertical L904
  constraint horizontal L918
  constraint vertical L914
  constraint horizontal L896
  constraint vertical L948
  constraint horizontal L949
  constraint vertical L913
  constraint horizontal L910
  constraint vertical L930
  constraint horizontal L995
  constraint vertical L938
  constraint horizontal L1033
  constraint vertical L1110
  constraint horizontal L1020
  constraint vertical L973
  constraint horizontal L1021
  constraint vertical L1012
  constraint horizontal L1013
  constraint vertical L894
  constraint horizontal L1025
  constraint vertical L1041
  constraint horizontal L1113
  constraint vertical L951
  constraint horizontal L1093
  constraint vertical L1034
  constraint horizontal L1108
  constraint vertical L916
  constraint horizontal L1100
  constraint vertical L1094
  constraint horizontal L1092
  constraint vertical L960
  constraint horizontal L1102
  constraint vertical L1101
  constraint horizontal L1109
  constraint vertical L1103
  constraint horizontal L1089
  constraint vertical L1115
  constraint horizontal L1039
  constraint vertical L1095
  constraint horizontal L1030
  constraint vertical L1053
  constraint horizontal L1031
  constraint vertical L1066
  constraint horizontal L1062
  constraint vertical L1019
  constraint horizontal L1067
  constraint vertical L1046
  constraint horizontal L1072
  constraint vertical L1114
  constraint horizontal L1097
  constraint vertical L1071
  constraint horizontal L885
  constraint vertical L852
  constraint horizontal L868
  constraint vertical L1112
  constraint horizontal L841
  constraint vertical L846
  constraint horizontal L847
  constraint vertical L1080
  constraint horizontal L861
  constraint vertical L853
  constraint horizontal L844
  constraint vertical L1049